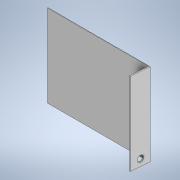
# Autodesk Inventor part: bottomCover
Saved by Autodesk Inventor 2020.3 (Build 243373000, 373)
## iProperties
Created: 2021-03-06
Part Number: bottomCover
Material: Generic
Document SubType Name: Modeling
Designer: allofus
Density: 1 g/cm^3
Appearance: Default
Author: allofus
Autodesk Inventor part; units mm, degrees
ref_plane "YZ Plane" through (0, 0, 0) normal (1, 0, 0) x (0, 1, 0)
ref_plane "XZ Plane" through (0, 0, 0) normal (0, 1, 0) x (-1, 0, 0)
ref_plane "XY Plane" through (0, 0, 0) normal (0, 0, 1) x (1, 0, 0)
sketch "Sketch1" plane through (0, 0, 0) normal (0, 1, 0) x (-1, 0, 0)
  line L0 (0, 0) -> (5, 0)
  line L1 (5, 161) -> (0, 161)
  line L2 (0, 0) -> (197.574, 0)
  line L3 (197.574, 0) -> (197.574, 1)
  line L4 (197.574, 1) -> (0, 1)
  line L5 (0, 1) -> (0, 0)
  line L6 (0, 1) -> (3.0069, 35.3687)
  line L7 (0, 1) -> (34.5, 1) construction
  line L8 (3.0069, 35.3687) -> (1.0145, 35.543)
  line L9 (1.0145, 35.543) -> (-2.0951, 0)
  line L10 (-2.0951, 0) -> (0, 0)
  line L11 (197.574, 1) -> (197.3061, 0)
  line L12 (197.574, 1) -> (198.6093, 1) construction
  line L13 (3.0069, 35.3687) -> (0.9992, 35.3687)
  dimension "d1" = 5
  dimension "d2" = 197.574
  dimension "d3" = 1
  dimension "d4" = 34.5
  dimension "d5" = 85
  dimension "d6" = 2
  dimension "d11" = 105
  constraints: 28 end point, 5 horizontal, 3 parallel, 3 perpendicular, 2 equal length, 2 point on line, 1 collinear
  measures "d1" distance of L1.start L1.end
  measures "d2" distance of L4.end L3.end
  measures "d3" distance of L3.end L2.end
  measures "d4" distance of L4.end L6.end
  measures "d5" angle of L7 L6
  measures "d6" distance of L6.end L8.end
  measures "d11" angle of L11 L12
extrude "Extrusion1" add sketch "Sketch1" along normal blind 161 contours L5 L4 L11 L2 L0 | L10 L9 L13 L6 L5 | L13 L9 L8
sketch "Sketch3" plane through (-3.0069, 0, 35.3687) normal (-0.9962, 0, -0.0872) x (-0.0872, 0, 0.9962)
  circle A0 centre (-17.9972, 13.5211) radius 6
  line L0 (-19.9848, 8.9507) -> (-15.1606, 8.9507)
  line L1 (-15.1606, 8.9507) -> (-15.1606, -1.5715)
  line L2 (-15.1606, -1.5715) -> (-19.9848, -1.5715)
  line L3 (-19.9848, -1.5715) -> (-19.9848, 8.9507)
  point P0 (-35.4962, 0)
  point P1 (-15.1606, 8.234)
  point P2 (-19.9848, 7.8599)
  dimension "d12" = 12
  constraints: 8 end point, 2 parallel, 1 centre point, 1 horizontal, 1 perpendicular
  measures "d12" diameter of A0
extrude "Extrusion3" cut sketch "Sketch3" against normal blind 58.2625 contours A0 L1 L0 L3 | L3 L0 L1 A0
body "Solid1"
